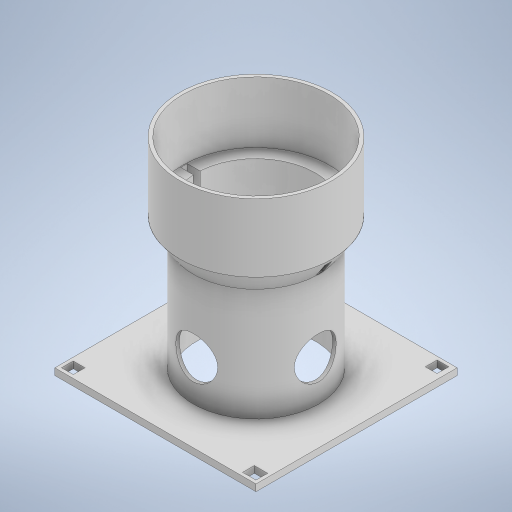
# Autodesk Inventor part: Stand
Saved by Autodesk Inventor 2023.2 (Build 272271030, 271C)
## iProperties
Created: 2023-04-02
Part Number: Stand
Material: Generic
Document SubType Name: Modeling
Designer: Lukas
Density: 1 g/cm^3
Appearance: Default
Author: Lukas
Autodesk Inventor part; units mm, degrees
ref_plane "Work Plane1" through (0, 83, 0) normal (0, 1, 0) x (1, 0, 0)
sketch "Sketch2" plane through (0, 83, 0) normal (0, 1, 0) x (1, 0, 0)
  circle A0 centre (0, 0) radius 43.55
  circle A1 centre (0, 0) radius 45.55
  circle A2 centre (0, 0) radius 35.45
  circle A3 centre (0, 0) radius 37.45
  dimension "d4" = 87.1
  dimension "d5" = 91.1
  dimension "d44" = 70.9
  dimension "d79" = 74.9
  constraints: 4 centre point, 4 coincident
  measures "d4" diameter of A0
  measures "d5" diameter of A1
  measures "d44" diameter of A2
  measures "d79" diameter of A3
extrude "Horni Cast" add sketch "Sketch2" along normal blind 36.5 contours A1
extrude "Spojka" add sketch "Sketch2" against normal blind 4 contours A0 | A1 | A3
extrude "Spodni Cast" add sketch "Sketch2" against normal blind 83 contours A3
ref_plane "Work Plane3" through (0, 0, 0) normal (0, -1, 0) x (1, 0, 0)
sketch "Sketch3" plane through (0, 0, 0) normal (0, -1, 0) x (1, 0, 0)
  circle A0 centre (0, 0) radius 35.45
  circle A1 centre (0, 0) radius 37.45
  line L0 (60, -60) -> (-60, -60)
  line L1 (-60, -60) -> (-60, 60)
  line L2 (-60, 60) -> (60, 60)
  line L3 (60, 60) -> (60, -60)
  line L4 (54, -54) -> (-54, -54)
  line L5 (-54, -54) -> (-54, 54)
  line L6 (-54, 54) -> (54, 54)
  line L7 (54, 54) -> (54, -54)
  circle A2 centre (0, 0) radius 45.55
  dimension "d14" = 70.9
  dimension "d15" = 74.9
  dimension "d22" = 60
  dimension "d23" = 60
  dimension "d24" = 60
  dimension "d25" = 60
  dimension "d28" = 6
  dimension "d29" = 6
  dimension "d30" = 6
  dimension "d31" = 6
  dimension "d46" = 91.1
  constraints: 16 end point, 4 parallel, 3 centre point, 3 coincident, 2 horizontal, 2 perpendicular
  measures "d14" diameter of A0
  measures "d15" diameter of A1
  measures "d22" distance from line of L3 point (0, 0)
  measures "d23" distance from line of L1 point (0, 0)
  measures "d24" distance from line of L2 point (0, 0)
  measures "d25" distance from line of L0 point (0, 0)
  measures "d28" distance between parallel lines of L4 L0
  measures "d29" distance between parallel lines of L3 L7
  measures "d30" distance between parallel lines of L1 L5
  measures "d31" distance between parallel lines of L6 L2
  measures "d46" diameter of A2
ref_plane "Work Plane4" through (0, -4, 0) normal (0, -1, 0) x (1, 0, 0)
ref_plane "Work Plane2" through (0, 83, 0) normal (0, 1, 0) x (1, 0, 0)
sketch "Sketch8" plane through (0, 0, 0) normal (1, 0, 0) x (0, 1, 0)
  circle A0 centre (24, 0) radius 12.5
  point P0 (0, 0)
  dimension "d64" = 25
  constraints: 1 centre point
  measures "d64" diameter of A0
extrude "DiryBok2" cut sketch "Sketch8" along normal mid plane 100
sketch "Sketch9" plane through (0, 0, 0) normal (0, 0, 1) x (1, 0, 0)
  circle A0 centre (0, 24) radius 12.5
  point P0 (0, 0)
  dimension "d67" = 25
  constraints: 1 centre point
  measures "d67" diameter of A0
extrude "DiryBok1" cut sketch "Sketch9" along normal mid plane 100
extrude "Malá Deska" add sketch "Sketch3" along normal blind 4 contours A1 | L0 L1 L2 L3 | L4 L5 L6 L7 | A2
sketch "Sketch10" plane through (0, 0, 0) normal (0, 1, 0) x (1, 0, 0)
  line L0 (-58, 58) -> (-51, 58)
  line L1 (-51, 58) -> (-51, 51)
  line L2 (-51, 51) -> (-58, 51)
  line L3 (-58, 51) -> (-58, 58)
  line L4 (-58, -58) -> (-51, -58)
  line L5 (-51, -58) -> (-51, -51)
  line L6 (-51, -51) -> (-58, -51)
  line L7 (-58, -51) -> (-58, -58)
  line L8 (58, -58) -> (50, -58)
  line L9 (50, -58) -> (50, -51)
  line L10 (50, -51) -> (58, -51)
  line L11 (58, -51) -> (58, -58)
  line L12 (50, 58) -> (57, 58)
  line L13 (57, 58) -> (57, 51)
  line L14 (57, 51) -> (50, 51)
  line L15 (50, 51) -> (50, 58)
  point P0 (0, 0)
  constraints: 32 end point, 8 parallel, 7 point on line, 4 horizontal, 4 perpendicular
extrude "Diry Deska" cut sketch "Sketch10" against normal blind 100
sketch "Sketch4" plane through (0, -4, 0) normal (0, -1, 0) x (1, 0, 0)
  line L0 (-94, -94) -> (94, -94) projected
  line L1 (94, -94) -> (84, -94)
  line L2 (84, -94) -> (84, -84)
  line L3 (84, -84) -> (94, -84)
  line L4 (94, -84) -> (94, -94)
  line L5 (94, 94) -> (-94, 94) projected
  line L6 (94, 94) -> (84, 94)
  line L7 (84, 94) -> (84, 84)
  line L8 (84, 84) -> (94, 84)
  line L9 (94, 84) -> (94, 94)
  line L10 (-94, -94) -> (-94, 94) projected
  line L11 (-94, 94) -> (-84, 94)
  line L12 (-84, 94) -> (-84, 84)
  line L13 (-84, 84) -> (-94, 84)
  line L14 (-94, 84) -> (-94, 94)
  line L15 (-94, -94) -> (-84, -94)
  line L16 (-84, -94) -> (-84, -84)
  line L17 (-84, -84) -> (-94, -84)
  line L18 (-94, -84) -> (-94, -94)
  line L19 (5, -94) -> (-5, -94)
  line L20 (-5, -94) -> (-5, -84)
  line L21 (-5, -84) -> (5, -84)
  line L22 (5, -84) -> (5, -94)
  line L23 (5, 94) -> (-5, 94)
  line L24 (-5, 94) -> (-5, 84)
  line L25 (-5, 84) -> (5, 84)
  line L26 (5, 84) -> (5, 94)
  line L27 (-94, -5) -> (-84, -5)
  line L28 (-84, -5) -> (-84, 5)
  line L29 (-84, 5) -> (-94, 5)
  line L30 (-94, 5) -> (-94, -5)
  line L31 (94, -94) -> (94, 94) projected
  line L32 (94, -5) -> (84, -5)
  line L33 (84, -5) -> (84, 5)
  line L34 (84, 5) -> (94, 5)
  line L35 (94, 5) -> (94, -5)
  point P0 (0, 0)
  constraints: 64 end point, 17 point on line, 16 parallel, 8 horizontal, 8 perpendicular
extrude "Nohy" [suppressed]
extrude "Velka Deska" [suppressed]
sketch "Sketch5" plane through (0, 83, 0) normal (0, 1, 0) x (1, 0, 0)
  line L0 (-35, 2) -> (-43, 2)
  line L1 (-43, 2) -> (-43, -2)
  line L2 (-43, -2) -> (-35, -2)
  line L3 (-35, -2) -> (-35, 2)
  line L4 (35, 2) -> (43, 2)
  line L5 (43, 2) -> (43, -2)
  line L6 (43, -2) -> (35, -2)
  line L7 (35, -2) -> (35, 2)
  line L8 (0, 55.58) -> (0, -55.58) projected
  point P0 (0, 0)
  dimension "d37" = 8
  dimension "d38" = 4
  dimension "d39" = 4
  dimension "d40" = 8
  dimension "d55" = 35
  dimension "d56" = 35
  constraints: 16 end point, 4 parallel, 2 horizontal, 2 perpendicular
  measures "d37" distance between parallel lines of L1 L3
  measures "d38" distance between parallel lines of L2 L0
  measures "d39" distance between parallel lines of L6 L4
  measures "d40" distance between parallel lines of L5 L7
  measures "d55" distance between parallel lines of L8 L7
  measures "d56" distance between parallel lines of L3 L8
chamfer "Chamfer2" distance 8 distance2 12 1 edges at (-37.45, 79, 0) measured on face at (42.5182, 79, -3.1568)
fillet "Fillet6" [suppressed]
extrude "Extrusion14" cut sketch "Sketch5" against normal blind 15
equation "\"d14\" = uzsi_prumer + gap"
equation "\"d34\" = vyska_nohy"
equation "\"d32\" = stand_vyska"
equation "\"d38\" = screw_headsize"
equation "\"d39\" = screw_headsize"
equation "\"stand_margin\" = 1"
equation "\"stand_vyska\" = 15"
equation "\"vyska_nohy\" = 100"
equation "\"screw_headsize\" = 4"
equation "\"screw_offset\" = 7.5"
equation "\"uzsi_prumer\" = 70.4"
equation "\"sirsi_prumer\" = 86.6"
equation "\"gap\" = 0.5"
equation "\"UpperTubeSize\" = 37.5"
body "Solid1"
